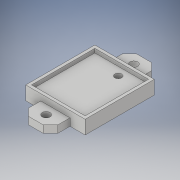
# Autodesk Inventor part: driver
Saved by Autodesk Inventor 2019.4 (Build 234330000, 330)
## iProperties
Created: 2020-04-10
Part Number: driver
Material: Типовые
Document SubType Name: Modeling
Designer: NoName
Density: 1 g/cm^3
Appearance: По умолчанию
Author: NoName
Autodesk Inventor part; units mm, degrees
ref_plane "YZ Plane" through (0, 0, 0) normal (1, 0, 0) x (0, 1, 0)
ref_plane "XZ Plane" through (0, 0, 0) normal (0, 1, 0) x (-1, 0, 0)
ref_plane "XY Plane" through (0, 0, 0) normal (0, 0, 1) x (1, 0, 0)
sketch "Эскиз1" plane through (0, 0, 0) normal (0, 1, 0) x (-1, 0, 0)
  line L0 (0, 14.2) -> (24.4, 14.2)
  line L1 (24.4, 14.2) -> (24.4, -14.2)
  line L2 (24.4, -14.2) -> (0, -14.2)
  line L3 (0, -14.2) -> (0, 0)
  line L4 (0, 0) -> (0, 14.2)
  point P0 (24.4, 0)
  dimension "d0" = 24.4
  dimension "d1" = 28.4
  constraints: 10 end point, 2 parallel, 1 horizontal, 1 horizontal alignment, 1 midpoint, 1 perpendicular, 1 vertical, 1 vertical alignment
  measures "d0" distance of L0.start L0.end
  measures "d1" distance between parallel lines of L2 L0
extrude "Выдавливание1" add sketch "Эскиз1" along normal blind 4
sketch "Эскиз2" plane through (0, 4, 0) normal (0, 1, 0) x (1, 0, 0)
  line L0 (-23.2, -13) -> (-1.2, -13)
  line L1 (-1.2, -13) -> (-1.2, 13)
  line L2 (-1.2, 13) -> (-23.2, 13)
  line L3 (-23.2, 13) -> (-23.2, -13)
  line L4 (0, 14.2) -> (-24.4, 14.2) projected
  line L5 (-24.4, 14.2) -> (-24.4, -14.2) projected
  line L6 (-24.4, -14.2) -> (0, -14.2) projected
  line L7 (0, -14.2) -> (0, 14.2) projected
  line L8 (0, 14.2) -> (-24.4, 14.2) projected
  line L9 (-24.4, 14.2) -> (-24.4, -14.2) projected
  point P0 (0, 0)
  point P1 (-12.2, 13)
  point P2 (-12.2, 14.2)
  point P3 (-23.2, 0)
  point P4 (-24.4, 0)
  dimension "d4" = 26
  dimension "d5" = 22
  constraints: 8 end point, 4 midpoint, 2 parallel, 1 horizontal, 1 horizontal alignment, 1 perpendicular, 1 vertical alignment
  measures "d4" distance of L2.end L0.start
  measures "d5" distance between parallel lines of L1 L3
extrude "Выдавливание2" add sketch "Эскиз2" along normal blind 1.6
sketch "Эскиз4" plane through (-24.4, 0, 14.2) normal (0, 0, 1) x (1, 0, 0)
  line L0 (6.2, 0) -> (18.2, 0)
  line L1 (18.2, 0) -> (18.2, 3)
  line L2 (18.2, 3) -> (6.2, 3)
  line L3 (6.2, 3) -> (6.2, 0)
  line L4 (0, 0) -> (24.4, 0) projected
  point P0 (12.2, 0)
  dimension "d8" = 3
  dimension "d9" = 12
  constraints: 8 end point, 2 midpoint, 2 parallel, 1 horizontal, 1 perpendicular
  measures "d8" distance between parallel lines of L0 L2
  measures "d9" distance between parallel lines of L3 L1
extrude "Выдавливание3" add sketch "Эскиз4" along normal blind 8
chamfer "Фаска1" distance 3 angle 45 2 edges at (-6.2, 1.5, 22.2) (-18.2, 1.5, 22.2)
mirror "Зеркальное отражение1" about plane through (0, 0, 0) normal (0, 0, 1) of "Выдавливание3", "Фаска1"
sketch "Эскиз6" plane through (-18.2, 3, 14.2) normal (0, 1, 0) x (1, 0, 0)
  line L0 (9, 36.4) -> (3, 36.4) projected
  line L1 (-5, 27.2) -> (-5, 1.2) projected
  line L2 (-5, 14.2) -> (17, 14.2)
  line L3 (17, 1.2) -> (17, 27.2) projected
  point P0 (18.2, 14.2)
  point P1 (6, -3.8)
  point P2 (6, 32.2)
  point P3 (6, 36.4)
  dimension "d23" = 36
  constraints: 3 midpoint, 2 end point, 2 vertical alignment, 1 symmetric about line
  measures "d23" distance of point (6, -3.8) point (6, 32.2)
hole "Отверстие1" at (-12.2, 3, 18) at (-12.2, 3, -18) direction (0, -1, 0) diameter 3.2 end through all
sketch "Эскиз7" plane through (0, 4, 0) normal (0, 1, 0) x (1, 0, 0)
  line L0 (-23.2, 13) -> (-1.2, 13) projected
  line L1 (-23.2, -13) -> (-23.2, 13) projected
  line L2 (-1.2, 13) -> (-1.2, -13) projected
  point P0 (0, 0)
  point P1 (-10.2, 9.6)
  dimension "d31" = 3.4
  dimension "d33" = 9
  measures "d31" distance from line of L0 point (-10.2, 9.6)
  measures "d33" distance from line of L2 point (-10.2, 9.6)
hole "Отверстие2" at (-10.2, 4, -9.6) direction (0, -1, 0) diameter 2.8 end through all
